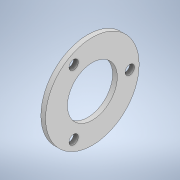
# Autodesk Inventor part: rodHolder
Saved by Autodesk Inventor 2020 (Build 240168000, 168)
## iProperties
Created: 2019-06-18
Part Number: rodHolder
Material: Generic
Document SubType Name: Modeling
Designer: Vivek Muskan
Density: 1 g/cm^3
Appearance: Default
Author: Vivek Muskan
Autodesk Inventor part; units mm, degrees
ref_plane "YZ Plane" through (0, 0, 0) normal (1, 0, 0) x (0, 1, 0)
ref_plane "XZ Plane" through (0, 0, 0) normal (0, 1, 0) x (-1, 0, 0)
ref_plane "XY Plane" through (0, 0, 0) normal (0, 0, 1) x (1, 0, 0)
sketch "Sketch1" plane through (0, 0, 0) normal (1, 0, 0) x (0, 1, 0)
  circle A0 centre (0, 0) radius 8
  line L0 (0, 0) -> (0, -12)
  circle A1 centre (0, -12) radius 1.5
  circle A2 centre (10.3923, 6) radius 1.5
  circle A3 centre (0, 0) radius 8
  circle A4 centre (-10.3923, 6) radius 1.5
  circle A5 centre (0, 0) radius 8
  circle A6 centre (0, 0) radius 15
  dimension "d0" = 16
  dimension "d1" = 12
  dimension "d2" = 3
  dimension "d5" = 360
  dimension "d7" = 30
  constraints: 7 centre point, 5 coincident, 2 end point, 1 vertical, 11 other
  measures "d0" diameter of A0
  measures "d1" distance of L0.start L0.end
  measures "d2" diameter of A1
  measures "d7" diameter of A6
extrude "Extrusion1" add sketch "Sketch1" along normal blind 1.5
body "Solid1"
